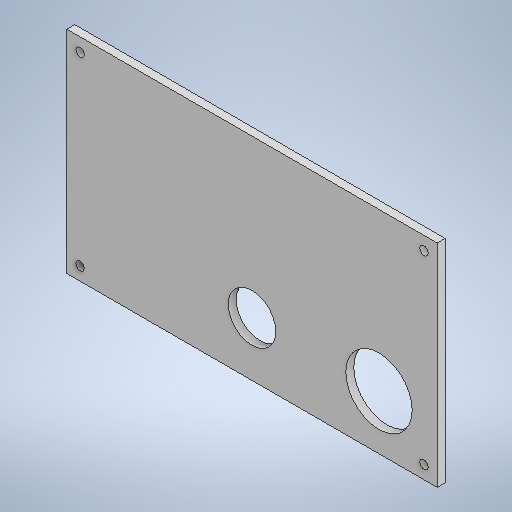
# Autodesk Inventor part: aaa_small_plate_middle
Saved by Autodesk Inventor 2025.1 (Build 291241000, 241)
## iProperties
Created: 2024-12-20
Part Number: aaa_small_plate_middle
Material: 一般
Document SubType Name: Modeling
Designer: yuki0520
Density: 1 g/cm^3
Appearance: 既定
Author: yuki0520
Autodesk Inventor part; units mm, degrees
ref_plane "YZ Plane" through (0, 0, 0) normal (1, 0, 0) x (0, 1, 0)
ref_plane "XZ Plane" through (0, 0, 0) normal (0, 1, 0) x (-1, 0, 0)
ref_plane "XY Plane" through (0, 0, 0) normal (0, 0, 1) x (1, 0, 0)
sketch "スケッチ1" plane through (0, 0, 0) normal (0, 0, 1) x (1, 0, 0)
  point P0 (0, 0)
sketch "スケッチ2" plane through (0, 0, 0) normal (0, 0, 1) x (1, 0, 0)
  line L0 (70, -40) -> (-70, -40)
  line L1 (-70, -40) -> (-70, 40)
  line L2 (-70, 40) -> (70, 40)
  line L3 (70, 40) -> (70, -40)
  line L4 (70, -40) -> (-70, 40) construction
  line L5 (-70, -40) -> (70, 40) construction
  circle A0 centre (-48, -19.5) radius 6.05
  circle A1 centre (48, -19.5) radius 12.55
  circle A2 centre (48, -19.5) radius 17.5
  circle A3 centre (65.5, -19.5) radius 2.05
  circle A4 centre (48, -2) radius 2.05
  circle A5 centre (30.5, -19.5) radius 2.05
  circle A6 centre (48, -37) radius 2.05
  circle A7 centre (-48, -19.5) radius 9
  circle A8 centre (-57, -19.5) radius 1.6
  circle A9 centre (-48, -28.5) radius 1.6
  circle A10 centre (-39, -19.5) radius 1.6
  circle A11 centre (-48, -10.5) radius 1.6
  line L6 (65, 35) -> (-65, 35)
  line L7 (-65, 35) -> (-65, -35)
  line L8 (-65, -35) -> (65, -35)
  line L9 (65, -35) -> (65, 35)
  line L10 (-65, 35) -> (-65, 35) construction
  line L11 (-66.6, 35) -> (-66.6, 35)
  line L12 (-63.4, 35) -> (-63.4, 35)
  arc A12 (-63.4, 35) -> (-66.6, 35) centre (-65, 35) ccw
  arc A13 (-66.6, 35) -> (-63.4, 35) centre (-65, 35) ccw
  line L13 (-65, 35) -> (-65, 35) construction
  line L14 (-65, -35) -> (-65, -35) construction
  line L15 (-63.4, -35) -> (-63.4, -35)
  line L16 (-66.6, -35) -> (-66.6, -35)
  arc A14 (-66.6, -35) -> (-63.4, -35) centre (-65, -35) ccw
  arc A15 (-63.4, -35) -> (-66.6, -35) centre (-65, -35) ccw
  line L17 (-65, -35) -> (-65, -35) construction
  line L18 (65, 35) -> (65, 35) construction
  line L19 (63.4, 35) -> (63.4, 35)
  line L20 (66.6, 35) -> (66.6, 35)
  arc A16 (66.6, 35) -> (63.4, 35) centre (65, 35) ccw
  arc A17 (63.4, 35) -> (66.6, 35) centre (65, 35) ccw
  line L21 (65, 35) -> (65, 35) construction
  line L22 (65, -35) -> (65, -35) construction
  line L23 (66.6, -35) -> (66.6, -35)
  line L24 (63.4, -35) -> (63.4, -35)
  arc A18 (63.4, -35) -> (66.6, -35) centre (65, -35) ccw
  arc A19 (66.6, -35) -> (63.4, -35) centre (65, -35) ccw
  line L25 (65, -35) -> (65, -35) construction
  line L26 (-70, -19.5) -> (70, -19.5)
  circle A20 centre (0, -19.5) radius 9
  circle A21 centre (0, -19.5) radius 39
  line L27 (-85, 40) -> (85, 40)
  line L28 (85, 40) -> (85, 35)
  line L29 (85, 35) -> (-85, 35)
  line L30 (-85, 35) -> (-85, 40)
  line L31 (-85, 35) -> (0, 0)
  line L32 (0, 0) -> (85, 35)
  line L33 (-70, 0) -> (70, 0)
  line L34 (70, 0) -> (70, -50)
  line L35 (70, -50) -> (-70, -50)
  line L36 (-70, -50) -> (-70, 0)
  point P0 (-65, -35)
  point P1 (65, 35)
  point P2 (65, -35)
  point P3 (-39.1422, -21.0937)
  point P4 (-39.1422, -17.9063)
  point P5 (0, 40)
  point P6 (85, 40)
  point P7 (48.45, -35)
  point P8 (47.55, -35)
  point P9 (-70, 28.8235)
  point P10 (70, 28.8235)
  dimension "d9" = 35
  dimension "d15" = 18
  dimension "d0" = 140
  dimension "d1" = 80
  dimension "d5" = 12.1
  dimension "d6" = 25.1
  dimension "d10" = 4.1
  dimension "d13" = 360
  dimension "d16" = 3.2
  dimension "d19" = 360
  dimension "d21" = 5
  dimension "d22" = 0
  dimension "d23" = 90
  dimension "d24" = 3.2
  dimension "d25" = 0
  dimension "d26" = 90
  dimension "d27" = 3.2
  dimension "d28" = 0
  dimension "d29" = 90
  dimension "d30" = 3.2
  dimension "d31" = 0
  dimension "d32" = 90
  dimension "d33" = 3.2
  dimension "d36" = 20.5
  dimension "d37" = 18
  dimension "d38" = 78
  dimension "d39" = 48
  dimension "d40" = 48
  dimension "d43" = 170
  dimension "d44" = 85
  dimension "d46" = 50
  constraints: 82 end point, 20 centre point, 16 point on circle, 16 tangent, 12 parallel, 9 midpoint, 9 perpendicular, 8 point on line, 7 horizontal, 5 collinear, 3 coincident, 1 horizontal alignment, 26 other
  measures "d0" distance of L1.end L2.end
  measures "d1" distance of L0.end L1.end
  measures "d5" diameter of A0
  measures "d6" diameter of A1
  measures "d10" diameter of A3
  measures "d16" diameter of A8
  measures "d21" distance between parallel lines of L2 L6
  measures "d22" distance of L6.end L10.end
  measures "d23" angle of L10 L13
  measures "d24" diameter of A13
  measures "d25" distance of L7.end L14.end
  measures "d26" angle of L17 L14
  measures "d27" diameter of A15
  measures "d28" distance of L6.start L18.end
  measures "d29" angle of L18 L21
  measures "d30" diameter of A17
  measures "d31" distance of L8.end L22.end
  measures "d32" angle of L25 L22
  measures "d33" diameter of A19
  measures "d36" distance between parallel lines of L0 L26
  measures "d37" diameter of A20
  measures "d38" diameter of A21
  measures "d39" distance of A1.centre A20.centre
  measures "d40" distance of A0.centre A20.centre
  measures "d43" distance of L28.end L29.end
  measures "d44" distance from line of point (0, 40) L30
  measures "d46" distance of L33.end L34.end
extrude "押し出し1" add sketch "スケッチ2" along normal blind 3 contours L0 A21 L8 A2 A6 A18 A19 L9 A3 L26 L3 | L0 A21 L8 | L26 A3 A2 L9 L33 L3 | L0 L1 L26 L7 A15 A14 L8 A21 | A21 A2 L8 | L8 A21 A10 L26 A20 A5 A2 | L33 L9 L32 L3 | L26 A2 A3 | A3 A2 L26 | L8 A15 L7 L26 A8 A7 A9 A10 A21 | L8 A6 A2 | A2 A21 A1 L26 A3 L9 L8 A6 | A2 A5 L26 A1 A21 | L32 L9 A17 L29 L3 | L33 A4 A21 L32 L9 | L9 A2 A4 L33 | A3 L9 A2 | A2 L26 L9 A3 | A3 L9 L26 A2 | A2 L9 A3 | L1 L33 L7 L26 | A21 L26 A10 | A10 A7 A21 | A6 L8 A2 | A2 A6 | A6 L8 | A5 L26 A2 | A2 L26 A5 | L29 A16 L6 A12 L1 L2 L3 | L32 A21 L31 L7 A13 L6 A17 L9 | L9 A3 L26 A1 A21 A2 A4 | L33 A4 | A4 A2 L33 | L9 L26 A3 | L9 A19 L8 A2 | A3 L26 L9 | L1 L31 L7 L33 | L7 L33 A21 A10 A7 A11 A8 L26 | A10 L26 A7 | A7 A9 A8 L26 A0 A10 | L26 A21 A10 | A10 A21 L33 A2 A5 L26 A20 | L26 A10 A7 | A7 A10 A21 | A6 L8 A2 | L26 A5 A2 | A2 A5 L26 | A5 A2 A21 A1 L26 | L32 L31 A21 | A21 L33 L32 | A4 A2 | A4 A2 A21 L33 | L1 L29 A13 L7 L31 | L7 L31 A21 L33 | L26 A7 A8 | A8 A7 L26 | A9 A7 | A7 A9 | L26 A0 A8 A7 A11 A10 | L31 L33 A21 | A8 L26 A7 | A7 L26 A8 | L26 A0 | A0 L26 | A11 A7 | A7 A11
equation "\"d27\" = d24"
equation "\"d30\" = d24"
equation "\"d33\" = d24"
equation "\"d40\" = d39"
equation "\"d44\" = 0.5 * d43"
